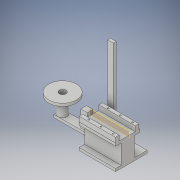
# Autodesk Inventor part: base
Saved by Autodesk Inventor 2018 (Build 220112000, 112)
## iProperties
Created: 2020-02-28
Part Number: base
Material: Generisch
Document SubType Name: Modeling
Designer: Tanja
Density: 1 g/cm^3
Appearance: Vorgabe
Author: Tanja
Autodesk Inventor part; units mm, degrees
ref_plane "YZ Plane" through (0, 0, 0) normal (1, 0, 0) x (0, 1, 0)
ref_plane "XZ Plane" through (0, 0, 0) normal (0, 1, 0) x (-1, 0, 0)
ref_plane "XY Plane" through (0, 0, 0) normal (0, 0, 1) x (1, 0, 0)
sketch "Skizze1" plane through (0, 0, 0) normal (0, 0, 1) x (1, 0, 0)
  line L0 (0, 0) -> (-75, 0)
  line L1 (-75, 0) -> (-75, 16)
  line L2 (-75, 16) -> (0, 16)
  line L3 (0, 16) -> (0, 0)
  dimension "d0" = 75
  dimension "d1" = 16
  constraints: 8 end point, 2 parallel, 1 horizontal, 1 perpendicular
  measures "d0" distance of L1.end L2.end
  measures "d1" distance of L0.end L1.end
extrude "Extrusion1" add sketch "Skizze1" along normal blind 5
sketch "Skizze2" plane through (0, 0, 5) normal (0, 0, 1) x (1, 0, 0)
  line L0 (0, 0) -> (0, 16) construction
  line L1 (-75, 0) -> (0, 0) construction
  line L2 (0, 0) -> (-75, 0) construction
  line L3 (-75, 0) -> (-75, 16) construction
  line L4 (-75, 16) -> (-75, 0) construction
  line L5 (-75, 16) -> (-59, 16) construction
  line L6 (-59, 16) -> (-59, 0) construction
  line L7 (-59, 16) -> (-75, 0) construction
  line L8 (-75, 16) -> (-59, 0) construction
  circle A0 centre (-67, 8) radius 8
  circle A1 centre (-67, 8) radius 6
  dimension "d4" = 16
  dimension "d5" = 16
  dimension "d6" = 16
  dimension "d7" = 12
  constraints: 12 end point, 2 centre point, 2 point on line, 1 coincident, 1 collinear, 1 midpoint, 1 perpendicular, 1 tangent
  measures "d4" distance of L1.start L3.end
  measures "d5" distance of L3.end L5.end
  measures "d6" distance of L5.end L6.end
  measures "d7" diameter of A1
extrude "Extrusion2" add sketch "Skizze2" along normal blind 30
sketch "Skizze3" plane through (-67, 8, 35) normal (0, 0, 1) x (1, 0, 0)
  circle A0 centre (0, 0) radius 6 construction
  line L0 (-6, 0) -> (6, 0) construction
  line L1 (0, 6) -> (0, -6) construction
  circle A1 centre (0, 0) radius 25
  circle A2 centre (0, 0) radius 6
  point P0 (67, -8)
  dimension "d10" = 50
  constraints: 4 end point, 4 point on circle, 2 coincident, 1 centre point, 1 horizontal, 1 perpendicular, 1 vertical alignment, 2 other
  measures "d10" diameter of A1
extrude "Extrusion4" add sketch "Skizze3" along normal blind 5
sketch "Skizze4" plane through (0, 0, 5) normal (0, 0, 1) x (1, 0, 0)
  circle A0 centre (-67, 8) radius 6 construction
  line L0 (-67, 8) -> (-17, 8) construction
  line L1 (-17, 8) -> (-17, 13) construction
  line L2 (-17, 13) -> (-29, 13) construction
  line L3 (-29, 13) -> (-29, 3) construction
  line L4 (-29, 3) -> (-17, 3)
  line L5 (-17, 3) -> (-17, 13)
  line L6 (-17, 13) -> (-29, 13)
  line L7 (-29, 13) -> (-29, 3)
  point P0 (0, 0)
  dimension "d15" = 50
  dimension "d16" = 5
  dimension "d17" = 12
  dimension "d18" = 10
  constraints: 16 end point, 3 perpendicular, 2 horizontal, 2 parallel, 1 vertical
  measures "d15" distance of L0.start L0.end
  measures "d16" distance of L0.end L1.end
  measures "d17" distance of L1.end L2.end
  measures "d18" distance of L2.end L3.end
extrude "Extrusion5" add sketch "Skizze4" along normal blind 30
sketch "Skizze5" plane through (0, 0, 5) normal (0, 0, 1) x (1, 0, 0)
  circle A0 centre (-67, 8) radius 6 construction
  line L0 (-67, 8) -> (0, 8) construction
  line L1 (0, 0) -> (0, 16) construction
  line L2 (0, 8) -> (0, -29) construction
  line L3 (0, -29) -> (66, -29) construction
  line L4 (0, 8) -> (0, 28) construction
  line L5 (66, -29) -> (0, -29)
  line L6 (0, -29) -> (0, 28)
  line L7 (0, 28) -> (66, 28)
  line L8 (66, 28) -> (66, -29)
  dimension "d21" = 67
  dimension "d22" = 37
  dimension "d23" = 66
  dimension "d24" = 20
  constraints: 16 end point, 2 horizontal, 2 parallel, 2 point on line, 1 midpoint, 1 perpendicular
  measures "d21" distance of L0.start L0.end
  measures "d22" distance of L0.end L2.end
  measures "d23" distance of L2.end L3.end
  measures "d24" distance of L0.end L4.end
extrude "Extrusion6" add sketch "Skizze5" against normal blind 5
sketch "Skizze6" plane through (0, 0, 5) normal (0, 0, 1) x (1, 0, 0)
  line L0 (0, -29) -> (0, 0) construction
  line L1 (0, -29) -> (0, 15) construction
  line L2 (0, 15) -> (66, 15) construction
  line L3 (66, 28) -> (66, -29) construction
  line L4 (0, 15) -> (0, 5) construction
  line L5 (66, -29) -> (0, -29) construction
  line L6 (66, -29) -> (66, -19) construction
  line L7 (0, 5) -> (66, 5)
  line L8 (66, 5) -> (66, -19)
  line L9 (66, -19) -> (0, -19)
  line L10 (0, -19) -> (0, 5)
  dimension "d27" = 44
  dimension "d28" = 66
  dimension "d42" = 10
  dimension "d43" = 10
  constraints: 16 end point, 3 point on line, 2 parallel, 1 collinear, 1 horizontal, 1 perpendicular
  measures "d27" distance of L0.start L1.end
  measures "d28" distance of L1.end L2.end
  measures "d42" distance of L1.end L4.end
  measures "d43" distance of L3.end L6.end
extrude "Extrusion7" add sketch "Skizze6" along normal blind 35
sketch "Skizze7" plane through (0, 0, 5) normal (0, 0, 1) x (1, 0, 0)
  line L0 (-67, 6.9194) -> (0, 7.5) construction
  line L1 (0, 0) -> (0, -19) construction
  line L2 (0, 7.5) -> (0, 22.5) construction
  line L3 (0, 22.5) -> (10, 22.5) construction
  line L4 (0, 28) -> (66, 28) projected
  line L5 (10, 22.5) -> (0, 22.5)
  line L6 (0, 22.5) -> (0, 28)
  line L7 (0, 28) -> (10, 28)
  line L8 (10, 28) -> (10, 22.5)
  point P0 (0, 15)
  dimension "d31" = 15
  dimension "d32" = 10
  constraints: 14 end point, 2 horizontal, 2 parallel, 1 collinear, 1 perpendicular, 1 point on line
  measures "d31" distance of L0.end L2.end
  measures "d32" distance of L2.end L3.end
extrude "Extrusion8" add sketch "Skizze7" along normal blind 143
sketch "Skizze9" plane through (0, 0, 40) normal (0, 0, 1) x (1, 0, 0)
  line L0 (0, 0) -> (0, 5) construction
  line L1 (0, 5) -> (0, 15) construction
  line L2 (0, 15) -> (66, 15) construction
  line L3 (66, 28) -> (66, -29) construction
  line L4 (66, 15) -> (66, -29) construction
  line L5 (66, -29) -> (0, -29) projected
  line L6 (0, 15) -> (66, 15)
  line L7 (66, 15) -> (66, -29)
  line L8 (66, -29) -> (0, -29)
  line L9 (0, -29) -> (0, 15)
  dimension "d44" = 10
  dimension "d45" = 66
  constraints: 14 end point, 2 parallel, 1 collinear, 1 horizontal, 1 perpendicular, 1 point on line, 1 vertical
  measures "d44" distance of L0.end L1.end
  measures "d45" distance of L1.end L2.end
extrude "Extrusion10" add sketch "Skizze9" along normal blind 5
sketch "Skizze10" plane through (0, 0, 45) normal (0, 0, 1) x (1, 0, 0)
  circle A0 centre (-67, 8) radius 6 construction
  line L0 (-67, 8) -> (0, 8) construction
  line L1 (0, 8) -> (0, -7) construction
  line L2 (0, 0) -> (0, 5) construction
  line L3 (0, -7) -> (0, 13.3) construction
  line L4 (0, 13.3) -> (66, 13.3) construction
  line L5 (66, 28) -> (66, -29) construction
  line L6 (66, 13.3) -> (66, 6.8) construction
  line L7 (66, 6.8) -> (0, 6.8) construction
  line L8 (66, 5) -> (0, 5) construction
  line L9 (66, 6.8) -> (132, 6.8) construction
  line L10 (0, 13.3) -> (0, 6.8) construction
  line L11 (0, 5) -> (0, 15) construction
  line L12 (0, 13.3) -> (66, 13.3)
  line L13 (66, 13.3) -> (66, 6.8)
  line L14 (66, 6.8) -> (0, 6.8)
  line L15 (0, 6.8) -> (0, 13.3)
  dimension "d48" = 15
  dimension "d49" = 20.3
  dimension "d50" = 66
  dimension "d51" = 6.5
  dimension "d52" = 66
  dimension "d53" = 180
  dimension "d54" = 6.5
  constraints: 24 end point, 3 collinear, 3 horizontal, 3 parallel, 3 point on line, 1 perpendicular
  measures "d48" distance of L0.end L1.end
  measures "d49" distance of L1.end L3.end
  measures "d50" distance of L3.end L4.end
  measures "d51" distance of L4.end L6.end
  measures "d52" distance of L6.end L7.end
  measures "d53" angle of L7 L9
  measures "d54" distance of L3.end L7.end
extrude "Extrusion11" add sketch "Skizze10" along normal blind 9
ref_plane "Arbeitsebene2" through (0, -7.9, 45) normal (0, -1, 0) x (1, 0, 0)
mirror "Spiegeln1" about plane through (0, -7.9, 45) normal (0, -1, 0) of "Extrusion11"
sketch "Skizze13" plane through (0, -29.1, 54) normal (0, 0, 1) x (1, 0, 0)
  circle A0 centre (14.0634, 3.7) radius 1.35 projected
  circle A1 centre (36.0634, 3.7) radius 1.35 projected
  circle A2 centre (58.0634, 3.7) radius 1.35 projected
  circle A3 centre (14.0634, 3.7) radius 1.4
  circle A4 centre (36.0634, 3.7) radius 1.4
  circle A5 centre (58.0634, 3.7) radius 1.4
  point P0 (0, 29.1)
  dimension "d58" = 2.8
  dimension "d59" = 2.8
  dimension "d60" = 2.8
  constraints: 3 centre point, 3 coincident
  measures "d58" diameter of A3
  measures "d59" diameter of A4
  measures "d60" diameter of A5
extrude "Extrusion12" cut sketch "Skizze13" against normal up to next contours A0 | A1 | A2 | A3 | A5
mirror "Spiegeln2" about plane through (0, -7.9, 45) normal (0, -1, 0) of "Extrusion12"
equation "\"d61\" = d60"
